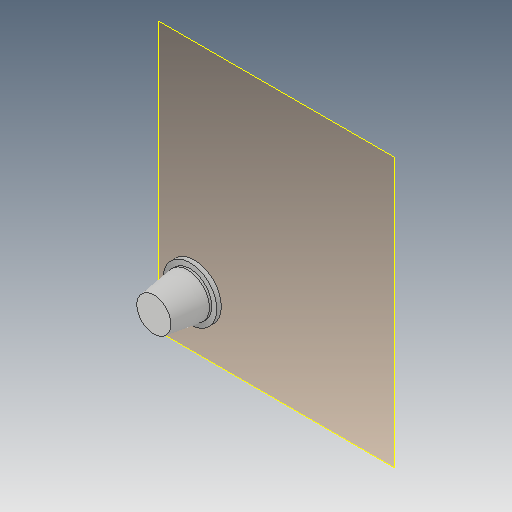
# Autodesk Inventor part: Knob
Saved by Autodesk Inventor 2017 (Build 210142000, 142)
## iProperties
Created: 2016-07-27
Part Number: Knob
Material: Generic
Document SubType Name: Modeling
Designer: User
Density: 1 g/cm^3
Appearance: Default
Mass: 4.70469 g
Surface Area: 18.1217 cm^2
Volume: 4.70469 cm^3
Author: User
Autodesk Inventor part; units mm, degrees
ref_plane "YZ Plane" through (0, 0, 0) normal (1, 0, 0) x (0, 1, 0)
ref_plane "XZ Plane" through (0, 0, 0) normal (0, 1, 0) x (-1, 0, 0)
ref_plane "XY Plane" through (0, 0, 0) normal (0, 0, 1) x (1, 0, 0)
sketch "Sketch1" plane through (0, 0, 0) normal (0, 0, 1) x (1, 0, 0)
  arc A0 (-34.8899, -33.6307) -> (-34.8899, -38.7172) centre (-36.3549, -36.1739) ccw projected
  circle A1 centre (-36.3549, -36.1739) radius 9.6697
  point P0 (0, 0)
  constraints: 1 centre point, 1 coincident
extrude "Extrusion1" add sketch "Sketch1" along normal blind 18
chamfer "Chamfer2" distance 15 angle 8 1 edges at (-46.0245, -36.1739, 18) measured on face at (-46.0245, -36.1739, 17.5)
ref_plane "Work Plane1" through (0, 0, 0) normal (0, 0, 1) x (1, 0, 0)
sketch "Sketch2" plane through (0, 0, 0) normal (0, 0, 1) x (1, 0, 0)
  circle A0 centre (-36.3549, -36.1739) radius 7.5616 projected
  circle A1 centre (-36.3549, -36.1739) radius 11.9385
  point P0 (0, 0)
  constraints: 1 centre point, 1 coincident
extrude "Extrusion2" add sketch "Sketch2" along normal blind 2
body "Solid1"
